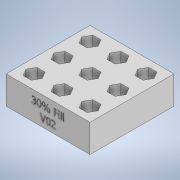
# Autodesk Inventor part: FootPad
Saved by Autodesk Inventor 2021.1 (Build 251245010, 245A)
## iProperties
Created: 2020-09-27
Part Number: FootPad
Material: Generic
Document SubType Name: Modeling
Designer: robst
Density: 1 g/cm^3
Appearance: Default
Author: robst
Autodesk Inventor part; units mm, degrees
ref_plane "YZ Plane" through (0, 0, 0) normal (1, 0, 0) x (0, 1, 0)
ref_plane "XZ Plane" through (0, 0, 0) normal (0, 1, 0) x (-1, 0, 0)
ref_plane "XY Plane" through (0, 0, 0) normal (0, 0, 1) x (1, 0, 0)
sketch "Sketch1" plane through (0, 0, 0) normal (0, 1, 0) x (-1, 0, 0)
  line L0 (-38.1, 38.1) -> (-38.1, -38.1)
  line L1 (-38.1, -38.1) -> (38.1, -38.1)
  line L2 (38.1, -38.1) -> (38.1, 38.1)
  line L3 (38.1, 38.1) -> (-38.1, 38.1)
  line L4 (-38.1, 38.1) -> (38.1, -38.1) construction
  line L5 (-38.1, -38.1) -> (38.1, 38.1) construction
  point P0 (0, 0)
  dimension "d0" = 76.2
  constraints: 12 end point, 2 midpoint, 2 parallel, 2 perpendicular, 1 vertical
  measures "d0" distance of L0.end L1.end
extrude "Extrusion1" add sketch "Sketch1" against normal blind 25.4
sketch "Sketch3" plane through (-38.1, 0, 38.1) normal (0, 0, 1) x (1, 0, 0)
  line L0 (0, 0) -> (0, -25.4) construction
  line L1 (0, -12.7) -> (76.2, -12.7) construction
  line L2 (76.2, 0) -> (76.2, -25.4) construction
  spline S0 degree 2 poles (25.1522, -5.658) (24.9299, -5.658) (24.4902, -5.7667) (24.2778, -5.8506) knots 0 0 0 1 2 2 2
  spline S1 degree 2 poles (24.2778, -5.8506) (24.0802, -5.9346) (23.7887, -6.1125) (23.6751, -6.1915) knots 0 0 0 1 2 2 2
  line L3 (23.6751, -6.1915) -> (23.6257, -6.1915)
  line L4 (23.6257, -6.1915) -> (23.6257, -5.327)
  spline S2 degree 2 poles (23.6257, -5.327) (23.8925, -5.1837) (24.8064, -4.9516) (25.2164, -4.9516) knots 0 0 0 1 2 2 2
  spline S3 degree 2 poles (25.2164, -4.9516) (25.6314, -4.9516) (26.2489, -5.1195) (26.5008, -5.2974) knots 0 0 0 1 2 2 2
  spline S4 degree 2 poles (26.5008, -5.2974) (26.7676, -5.49) (27.0442, -6.0482) (27.0442, -6.4237) knots 0 0 0 1 2 2 2
  spline S5 degree 2 poles (27.0442, -6.4237) (27.0442, -6.9276) (26.3822, -7.6883) (25.9179, -7.7871) knots 0 0 0 1 2 2 2
  line L5 (25.9179, -7.7871) -> (25.9179, -7.8464)
  spline S6 degree 2 poles (25.9179, -7.8464) (26.1105, -7.8859) (26.5502, -8.0638) (26.7379, -8.2416) knots 0 0 0 1 2 2 2
  spline S7 degree 2 poles (26.7379, -8.2416) (26.9256, -8.4145) (27.1628, -8.9678) (27.1628, -9.3679) knots 0 0 0 1 2 2 2
  spline S8 degree 2 poles (27.1628, -9.3679) (27.1628, -9.778) (26.8812, -10.4745) (26.6243, -10.7413) knots 0 0 0 1 2 2 2
  spline S9 degree 2 poles (26.6243, -10.7413) (26.3575, -11.0179) (25.6017, -11.3044) (25.1225, -11.3044) knots 0 0 0 1 2 2 2
  spline S10 degree 2 poles (25.1225, -11.3044) (24.6631, -11.3044) (23.764, -11.0821) (23.4577, -10.929) knots 0 0 0 1 2 2 2
  line L6 (23.4577, -10.929) -> (23.4577, -10.0645)
  line L7 (23.4577, -10.0645) -> (23.517, -10.0645)
  spline S11 degree 2 poles (23.517, -10.0645) (23.7739, -10.2522) (24.6434, -10.598) (25.0731, -10.598) knots 0 0 0 1 2 2 2
  spline S12 degree 2 poles (25.0731, -10.598) (25.3251, -10.598) (25.829, -10.4399) (25.9969, -10.2572) knots 0 0 0 1 2 2 2
  spline S13 degree 2 poles (25.9969, -10.2572) (26.1599, -10.0744) (26.3328, -9.6396) (26.3328, -9.3087) knots 0 0 0 1 2 2 2
  spline S14 degree 2 poles (26.3328, -9.3087) (26.3328, -8.9777) (26.1402, -8.5479) (25.9673, -8.4244) knots 0 0 0 1 2 2 2
  spline S15 degree 2 poles (25.9673, -8.4244) (25.7944, -8.3009) (25.3251, -8.207) (25.0484, -8.207) knots 0 0 0 1 2 2 2
  line L8 (25.0484, -8.207) -> (24.7026, -8.207)
  line L9 (24.7026, -8.207) -> (24.7026, -7.5303)
  line L10 (24.7026, -7.5303) -> (24.9743, -7.5303)
  spline S16 degree 2 poles (24.9743, -7.5303) (25.5227, -7.5303) (26.2143, -7.0066) (26.2143, -6.5077) knots 0 0 0 1 2 2 2
  spline S17 degree 2 poles (26.2143, -6.5077) (26.2143, -6.2755) (26.0364, -5.9445) (25.8932, -5.8457) knots 0 0 0 1 2 2 2
  spline S18 degree 2 poles (25.8932, -5.8457) (25.74, -5.742) (25.3646, -5.658) (25.1522, -5.658) knots 0 0 0 1 2 2 2
  spline S19 degree 2 poles (31.8756, -8.128) (31.8756, -9.7681) (30.9221, -11.3044) (29.9292, -11.3044) knots 0 0 0 1 2 2 2
  spline S20 degree 2 poles (29.9292, -11.3044) (28.9214, -11.3044) (27.9779, -9.7385) (27.9779, -8.1329) knots 0 0 0 1 2 2 2
  spline S21 degree 2 poles (27.9779, -8.1329) (27.9779, -6.483) (28.9313, -4.9565) (29.9292, -4.9565) knots 0 0 0 1 2 2 2
  spline S22 degree 2 poles (29.9292, -4.9565) (30.932, -4.9565) (31.8756, -6.5373) (31.8756, -8.128) knots 0 0 0 1 2 2 2
  spline S23 degree 2 poles (30.8283, -9.9855) (30.9468, -9.6841) (31.0456, -8.7554) (31.0456, -8.128) knots 0 0 0 1 2 2 2
  spline S24 degree 2 poles (31.0456, -8.128) (31.0456, -7.5006) (30.9468, -6.5768) (30.8233, -6.2656) knots 0 0 0 1 2 2 2
  spline S25 degree 2 poles (30.8233, -6.2656) (30.6998, -5.9544) (30.27, -5.6333) (29.9292, -5.6333) knots 0 0 0 1 2 2 2
  spline S26 degree 2 poles (29.9292, -5.6333) (29.5883, -5.6333) (29.1487, -5.9544) (29.0202, -6.2755) knots 0 0 0 1 2 2 2
  spline S27 degree 2 poles (29.0202, -6.2755) (28.8967, -6.5867) (28.8078, -7.5352) (28.8078, -8.1329) knots 0 0 0 1 2 2 2
  spline S28 degree 2 poles (28.8078, -8.1329) (28.8078, -8.7751) (28.8868, -9.6347) (29.0153, -9.9706) knots 0 0 0 1 2 2 2
  spline S29 degree 2 poles (29.0153, -9.9706) (29.1338, -10.2868) (29.5735, -10.6277) (29.9292, -10.6277) knots 0 0 0 1 2 2 2
  spline S30 degree 2 poles (29.9292, -10.6277) (30.2651, -10.6277) (30.7048, -10.3066) (30.8283, -9.9855) knots 0 0 0 1 2 2 2
  spline S31 degree 2 poles (39.9772, -9.4865) (39.9772, -10.4054) (39.2362, -11.2946) (38.5347, -11.2946) knots 0 0 0 1 2 2 2
  spline S32 degree 2 poles (38.5347, -11.2946) (37.8234, -11.2946) (37.0922, -10.3955) (37.0922, -9.4865) knots 0 0 0 1 2 2 2
  spline S33 degree 2 poles (37.0922, -9.4865) (37.0922, -8.5726) (37.8382, -7.6785) (38.5347, -7.6785) knots 0 0 0 1 2 2 2
  spline S34 degree 2 poles (38.5347, -7.6785) (39.251, -7.6785) (39.9772, -8.5775) (39.9772, -9.4865) knots 0 0 0 1 2 2 2
  spline S35 degree 2 poles (35.5164, -6.7744) (35.5164, -7.6933) (34.7754, -8.5825) (34.0739, -8.5825) knots 0 0 0 1 2 2 2
  spline S36 degree 2 poles (34.0739, -8.5825) (33.3625, -8.5825) (32.6314, -7.6834) (32.6314, -6.7744) knots 0 0 0 1 2 2 2
  spline S37 degree 2 poles (32.6314, -6.7744) (32.6314, -5.8605) (33.3773, -4.9664) (34.0739, -4.9664) knots 0 0 0 1 2 2 2
  spline S38 degree 2 poles (34.0739, -4.9664) (34.7902, -4.9664) (35.5164, -5.8655) (35.5164, -6.7744) knots 0 0 0 1 2 2 2
  line L11 (38.2433, -5.08) -> (35.052, -11.176)
  line L12 (35.052, -11.176) -> (34.3752, -11.176)
  line L13 (34.3752, -11.176) -> (37.5665, -5.08)
  line L14 (37.5665, -5.08) -> (38.2433, -5.08)
  spline S39 degree 2 poles (39.251, -9.4865) (39.251, -8.8591) (38.9596, -8.2219) (38.5397, -8.2219) knots 0 0 0 1 2 2 2
  spline S40 degree 2 poles (38.5397, -8.2219) (38.1198, -8.2219) (37.8234, -8.869) (37.8234, -9.4865) knots 0 0 0 1 2 2 2
  spline S41 degree 2 poles (37.8234, -9.4865) (37.8234, -10.104) (38.1, -10.7512) (38.5397, -10.7512) knots 0 0 0 1 2 2 2
  spline S42 degree 2 poles (38.5397, -10.7512) (38.9596, -10.7512) (39.251, -10.104) (39.251, -9.4865) knots 0 0 0 1 2 2 2
  spline S43 degree 2 poles (34.7902, -6.7744) (34.7902, -6.147) (34.4987, -5.5098) (34.0788, -5.5098) knots 0 0 0 1 2 2 2
  spline S44 degree 2 poles (34.0788, -5.5098) (33.6589, -5.5098) (33.3625, -6.1569) (33.3625, -6.7744) knots 0 0 0 1 2 2 2
  spline S45 degree 2 poles (33.3625, -6.7744) (33.3625, -7.3919) (33.6392, -8.0391) (34.0788, -8.0391) knots 0 0 0 1 2 2 2
  spline S46 degree 2 poles (34.0788, -8.0391) (34.4987, -8.0391) (34.7902, -7.3919) (34.7902, -6.7744) knots 0 0 0 1 2 2 2
  line L15 (47.2786, -5.8012) -> (44.443, -5.8012)
  line L16 (44.443, -5.8012) -> (44.443, -7.5204)
  line L17 (44.443, -7.5204) -> (47.16, -7.5204)
  line L18 (47.16, -7.5204) -> (47.16, -8.2416)
  line L19 (47.16, -8.2416) -> (44.443, -8.2416)
  line L20 (44.443, -8.2416) -> (44.443, -11.176)
  line L21 (44.443, -11.176) -> (43.6328, -11.176)
  line L22 (43.6328, -11.176) -> (43.6328, -5.08)
  line L23 (43.6328, -5.08) -> (47.2786, -5.08)
  line L24 (47.2786, -5.08) -> (47.2786, -5.8012)
  line L25 (48.7309, -11.176) -> (47.9603, -11.176)
  line L26 (47.9603, -11.176) -> (47.9603, -6.6015)
  line L27 (47.9603, -6.6015) -> (48.7309, -6.6015)
  line L28 (48.7309, -6.6015) -> (48.7309, -11.176)
  line L29 (48.7853, -5.8408) -> (47.9109, -5.8408)
  line L30 (47.9109, -5.8408) -> (47.9109, -5.0405)
  line L31 (47.9109, -5.0405) -> (48.7853, -5.0405)
  line L32 (48.7853, -5.0405) -> (48.7853, -5.8408)
  line L33 (50.6477, -11.176) -> (49.877, -11.176)
  line L34 (49.877, -11.176) -> (49.877, -4.8083)
  line L35 (49.877, -4.8083) -> (50.6477, -4.8083)
  line L36 (50.6477, -4.8083) -> (50.6477, -11.176)
  line L37 (52.5644, -11.176) -> (51.7938, -11.176)
  line L38 (51.7938, -11.176) -> (51.7938, -4.8083)
  line L39 (51.7938, -4.8083) -> (52.5644, -4.8083)
  line L40 (52.5644, -4.8083) -> (52.5644, -11.176)
  line L41 (36.0622, -15.1467) -> (33.9627, -21.2427)
  line L42 (33.9627, -21.2427) -> (33.0883, -21.2427)
  line L43 (33.0883, -21.2427) -> (30.9888, -15.1467)
  line L44 (30.9888, -15.1467) -> (31.8583, -15.1467)
  line L45 (31.8583, -15.1467) -> (33.5478, -20.2102)
  line L46 (33.5478, -20.2102) -> (35.2373, -15.1467)
  line L47 (35.2373, -15.1467) -> (36.0622, -15.1467)
  spline S47 degree 2 poles (40.3354, -18.1947) (40.3354, -19.8348) (39.3819, -21.3711) (38.389, -21.3711) knots 0 0 0 1 2 2 2
  spline S48 degree 2 poles (38.389, -21.3711) (37.3812, -21.3711) (36.4377, -19.8051) (36.4377, -18.1996) knots 0 0 0 1 2 2 2
  spline S49 degree 2 poles (36.4377, -18.1996) (36.4377, -16.5497) (37.3911, -15.0232) (38.389, -15.0232) knots 0 0 0 1 2 2 2
  spline S50 degree 2 poles (38.389, -15.0232) (39.3918, -15.0232) (40.3354, -16.604) (40.3354, -18.1947) knots 0 0 0 1 2 2 2
  spline S51 degree 2 poles (39.2881, -20.0521) (39.4066, -19.7508) (39.5054, -18.8221) (39.5054, -18.1947) knots 0 0 0 1 2 2 2
  spline S52 degree 2 poles (39.5054, -18.1947) (39.5054, -17.5673) (39.4066, -16.6435) (39.2831, -16.3323) knots 0 0 0 1 2 2 2
  spline S53 degree 2 poles (39.2831, -16.3323) (39.1596, -16.0211) (38.7299, -15.7) (38.389, -15.7) knots 0 0 0 1 2 2 2
  spline S54 degree 2 poles (38.389, -15.7) (38.0481, -15.7) (37.6085, -16.0211) (37.48, -16.3422) knots 0 0 0 1 2 2 2
  spline S55 degree 2 poles (37.48, -16.3422) (37.3565, -16.6534) (37.2676, -17.6019) (37.2676, -18.1996) knots 0 0 0 1 2 2 2
  spline S56 degree 2 poles (37.2676, -18.1996) (37.2676, -18.8418) (37.3466, -19.7014) (37.4751, -20.0373) knots 0 0 0 1 2 2 2
  spline S57 degree 2 poles (37.4751, -20.0373) (37.5936, -20.3535) (38.0333, -20.6943) (38.389, -20.6943) knots 0 0 0 1 2 2 2
  spline S58 degree 2 poles (38.389, -20.6943) (38.7249, -20.6943) (39.1646, -20.3732) (39.2881, -20.0521) knots 0 0 0 1 2 2 2
  line L48 (44.8753, -21.2427) -> (41.1159, -21.2427)
  line L49 (41.1159, -21.2427) -> (41.1159, -20.3782)
  spline S59 degree 2 poles (41.1159, -20.3782) (41.521, -19.9978) (42.2422, -19.2914) (42.588, -18.911) knots 0 0 0 1 2 2 2
  spline S60 degree 2 poles (42.588, -18.911) (43.2846, -18.1453) (43.7934, -17.2264) (43.7934, -16.7374) knots 0 0 0 1 2 2 2
  spline S61 degree 2 poles (43.7934, -16.7374) (43.7934, -16.4805) (43.6353, -16.0952) (43.492, -15.9717) knots 0 0 0 1 2 2 2
  spline S62 degree 2 poles (43.492, -15.9717) (43.3488, -15.8482) (42.9733, -15.7247) (42.7461, -15.7247) knots 0 0 0 1 2 2 2
  spline S63 degree 2 poles (42.7461, -15.7247) (42.5287, -15.7247) (42.0841, -15.8334) (41.8816, -15.9173) knots 0 0 0 1 2 2 2
  spline S64 degree 2 poles (41.8816, -15.9173) (41.7087, -15.9865) (41.3876, -16.1841) (41.2888, -16.2533) knots 0 0 0 1 2 2 2
  line L50 (41.2888, -16.2533) -> (41.2443, -16.2533)
  line L51 (41.2443, -16.2533) -> (41.2443, -15.3838)
  spline S65 degree 2 poles (41.2443, -15.3838) (41.4963, -15.2603) (42.4003, -15.0182) (42.8054, -15.0182) knots 0 0 0 1 2 2 2
  spline S66 degree 2 poles (42.8054, -15.0182) (43.66, -15.0182) (44.6233, -15.9223) (44.6233, -16.6929) knots 0 0 0 1 2 2 2
  spline S67 degree 2 poles (44.6233, -16.6929) (44.6233, -17.0535) (44.4554, -17.6562) (44.3072, -17.9131) knots 0 0 0 1 2 2 2
  spline S68 degree 2 poles (44.3072, -17.9131) (44.1589, -18.1799) (43.7292, -18.7035) (43.492, -18.9555) knots 0 0 0 1 2 2 2
  spline S69 degree 2 poles (43.492, -18.9555) (43.1067, -19.3754) (42.1632, -20.2744) (41.8816, -20.5363) knots 0 0 0 1 2 2 2
  line L52 (41.8816, -20.5363) -> (44.8753, -20.5363)
  line L53 (44.8753, -20.5363) -> (44.8753, -21.2427)
  point P0 (38.1, 0)
  constraints: 2 end point, 2 midpoint, 1 horizontal
extrude "Extrusion3" cut sketch "Sketch3" against normal blind 1.27
sketch "Sketch2" plane through (0, 0, 0) normal (0, 1, 0) x (1, 0, 0)
  line L0 (-38.1, -38.1) -> (38.1, -38.1) projected
  line L1 (38.1, -38.1) -> (38.1, 38.1) projected
  line L2 (29.0662, -19.05) -> (32.7323, -25.4)
  line L3 (32.7323, -25.4) -> (29.0662, -31.75)
  line L4 (29.0662, -31.75) -> (21.7338, -31.75)
  line L5 (21.7338, -31.75) -> (18.0677, -25.4)
  line L6 (18.0677, -25.4) -> (21.7338, -19.05)
  line L7 (21.7338, -19.05) -> (29.0662, -19.05)
  line L8 (38.1, 38.1) -> (-38.1, 38.1) projected
  point P0 (0, 0)
  point P1 (25.4, -25.4)
  dimension "d16" = 12.7
  dimension "d17" = 12.7
  dimension "d18" = 12.7
  constraints: 12 end point, 1 parallel, 13 other
  measures "d16" distance between parallel lines of L4 L7
  measures "d17" distance from line of L0 point (25.4, -25.4)
  measures "d18" distance from line of L1 point (25.4, -25.4)
extrude "Extrusion2" cut sketch "Sketch2" against normal through all
pattern_linear "Rectangular Pattern1" count 3 spacing 25.4 along (-1, 0, 0) count 3 spacing 25.4 along (0, 0, -1) of "Extrusion2"
equation "\"d0\" = width"
equation "\"d1\" = height"
equation "\"width\" = 76.2"
equation "\"height\" = 25.4"
equation "\"holeDiameter\" = 12.7"
body "Solid1"
